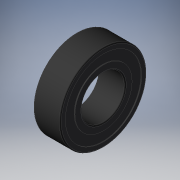
# Autodesk Inventor part: bearing_688
Saved by Autodesk Inventor 2019 (Build 230136000, 136)
## iProperties
Created: 2023-11-09
Part Number: bearing_688
Material: Generic
Catalog Web Link: www.cadenas.de
Description: 600_bearing-Small Ball Bearings
Vendor: MISUMI
Document SubType Name: Modeling
Designer: psAdmin
Manufacturer: MISUMI
Mass: 0.730663 g
Surface Area: 6.90443 cm^2
Volume: 0.730663 cm^3
Density: 1 g/cm^3
Appearance: PSOLRGB-175-175-175
Category: PARTsolutions
Company: MISUMI
Title: bearing_688
Author: Cadenas PARTsolutions
Comments: Small Ball Bearings
PSOL_IDENT_0: {$CADENAS_DATA/23d-libs/misumi/metric/accessories/bearing_600.prj},168 {VTYP=3D},{NB=bearing_688},{L
PSOL_IDENT_1: INA=bearing_688},{NN=600_bearing},{DATE=08.06.2021 06:39:28},{GEOMDATE=24.10.2013 00:00:00},{VERSION=
PSOL_IDENT_2: },{LINEID=270},{WBVAR=},{WBNUMERIC=}  {NB=bearing_688},{LINA=bearing_688},{KT=DUMMY},{PN=bearing_688
PSOL_IDENT_3: },{BN=688},{DD=8.0},{D=16},{B=5.0},{RR=0.20},{DS=9.60},{DDHH=14.40},{R=0.20},{MASS=4.02},{A=4.6800},
PSOL_IDENT_4: {C=1.280},{BB=0.944}
NB: bearing_688
NN: 600_bearing
NT: Small Ball Bearings
NBSYN: $PN.
LINA: bearing_688
CATALOG: Misumi
PN: bearing_688
BN: 688
DD: 8
D: 16
B: 5
RR: 0.2
DS: 9.6
DDHH: 14.4
R: 0.2
MASS: 4.02
SUPPLIER: MISUMI
ARTICLENO: bearing_688
BOMINFO: bearing_688
CREATOR: CADENAS GmbH
Autodesk Inventor part; units mm, degrees
sketch "Sketch_1" plane through (0, 0, 0) normal (0, 0, 1) x (1, 0, 0)
  line L0 (4.8, 0) -> (0.2, 0)
  arc A0 (0, 4.2) -> (0.2, 4) centre (0.2, 4.2) ccw
  line L1 (0.2, 4) -> (4.8, 4)
  arc A1 (4.8, 4) -> (5, 4.2) centre (4.8, 4.2) ccw
  line L2 (5, 4.2) -> (5, 5.28)
  line L3 (5, 5.28) -> (4.84, 5.28)
  line L4 (4.84, 5.28) -> (4.84, 7.056)
  line L5 (4.84, 7.056) -> (5, 7.056)
  line L6 (5, 7.056) -> (5, 7.8)
  arc A2 (5, 7.8) -> (4.8, 8) centre (4.8, 7.8) ccw
  line L7 (4.8, 8) -> (0.2, 8)
  arc A3 (0.2, 8) -> (0, 7.8) centre (0.2, 7.8) ccw
  line L8 (0, 7.8) -> (0, 7.056)
  line L9 (0, 7.056) -> (0.16, 7.056)
  line L10 (0.16, 7.056) -> (0.16, 5.28)
  line L11 (0.16, 5.28) -> (0, 5.28)
  line L12 (0, 5.28) -> (0, 4.2)
  constraints: 26 end point, 8 point on circle, 4 centre point
revolve "Revolution1" add sketch "Sketch_1" angle 360 about axis through (4.8, 0, 0) along (1, 0, 0)
ref_plane "to_housing_XY" through (0, 0, 0) normal (1, 0, 0) x (0, 0, -1)
ref_plane "to_housing_YZ" through (0, 0, 0) normal (0, 0, -1) x (0, 1, 0)
ref_plane "to_housing_ZX" through (0, 0, 0) normal (0, 1, 0) x (1, 0, 0)
ref_plane "to_housing_center_XY" through (2.5, 0, 0) normal (1, 0, 0) x (0, 0, -1)
ref_plane "to_housing_center_YZ" through (2.5, 0, 0) normal (0, 0, -1) x (0, 1, 0)
ref_plane "to_housing_center_ZX" through (2.5, 0, 0) normal (0, 1, 0) x (1, 0, 0)
body "Solid1"
